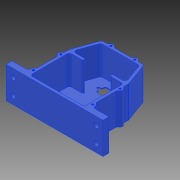
# Autodesk Inventor part: Cam.case.Back
Saved by Autodesk Inventor 2011 (Build 150239000, 239)
## iProperties
Created: 2011-03-29
Part Number: Cam.case.Back
Document SubType Name: Modeling
Designer: Rob
Density: 2.71 g/cm^3
Material: Aluminum-6061
Mass: 146.728 g
Surface Area: 368.166 cm^2
Volume: 54.143 cm^3
Author: Rob
Autodesk Inventor part; units mm, degrees
ref_plane "YZ Plane" through (0, 0, 0) normal (1, 0, 0) x (0, 1, 0)
ref_plane "XZ Plane" through (0, 0, 0) normal (0, 1, 0) x (-1, 0, 0)
ref_plane "XY Plane" through (0, 0, 0) normal (0, 0, 1) x (1, 0, 0)
sketch "Sketch1" plane through (0, 0, 0) normal (0, 0, 1) x (1, 0, 0)
  line L0 (0, 0) -> (0, 80.3)
  line L1 (-56.81, 0) -> (-56.81, 7)
  line L2 (-56.81, 7) -> (-34.81, 7)
  line L3 (0, 0) -> (-56.81, 0)
  line L4 (-34.81, 7) -> (-34.81, 52.2)
  line L5 (0, 80.3) -> (-24.7, 80.3)
  line L6 (-24.7, 80.3) -> (-34.81, 52.2)
  line L7 (0, 77.3) -> (-22.5911, 77.3)
  line L8 (-31.6217, 52.2) -> (-22.5911, 77.3)
  line L9 (-31.6217, 52.2) -> (0, 52.2)
  line L10 (-31.81, 49.2) -> (-31.81, 3)
  line L11 (0, 49.2) -> (-31.81, 49.2)
  line L12 (0, 3) -> (-31.81, 3)
  line L13 (56.81, 0) -> (56.81, 7)
  line L14 (56.81, 7) -> (34.81, 7)
  line L15 (0, 0) -> (56.81, 0)
  line L16 (34.81, 7) -> (34.81, 52.2)
  line L17 (0, 80.3) -> (24.7, 80.3)
  line L18 (24.7, 80.3) -> (34.81, 52.2)
  line L19 (0, 77.3) -> (22.5911, 77.3)
  line L20 (31.6217, 52.2) -> (22.5911, 77.3)
  line L21 (31.6217, 52.2) -> (0, 52.2)
  line L22 (31.81, 49.2) -> (31.81, 3)
  line L23 (0, 49.2) -> (31.81, 49.2)
  line L24 (0, 3) -> (31.81, 3)
  circle A0 centre (-34.81, 10) radius 3
  circle A1 centre (-34.81, 42.2) radius 3
  circle A2 centre (34.81, 42.2) radius 3
  circle A3 centre (34.81, 10) radius 3
  circle A4 centre (-14, 80.3) radius 3
  circle A5 centre (14, 80.3) radius 3
  dimension "d2" = 7
  dimension "d3" = 22
  dimension "d5" = 45.2
  dimension "d6" = 56.81
  dimension "d7" = 24.7
  dimension "d8" = 28.1
  dimension "d10" = 3
  dimension "d12" = 3
  dimension "d13" = 25.1
  dimension "d14" = 3
  dimension "d15" = 3
  dimension "d16" = 3
  dimension "d19" = 6
  dimension "d20" = 6
  dimension "d21" = 6
  dimension "d22" = 6
  dimension "d23" = 10
  dimension "d24" = 10
  dimension "d25" = 10
  dimension "d26" = 10
  dimension "d27" = 6
  dimension "d28" = 6
  dimension "d29" = 14
  dimension "d30" = 14
  constraints: 52 end point, 10 point on line, 9 symmetric about line, 6 centre point, 6 perpendicular, 5 parallel, 1 vertical
  measures "d2" distance of L1.start L1.end
  measures "d3" distance of L1.end L2.end
  measures "d5" distance of L2.end L4.end
  measures "d6" distance of L0.start L1.start
  measures "d7" distance of L0.end L5.end
  measures "d8" vertical distance of L5.end L4.end
  measures "d10" distance between parallel lines of L5 L7
  measures "d12" distance between parallel lines of L6 L8
  measures "d13" distance between parallel lines of L7 L9
  measures "d14" distance between parallel lines of L11 L9
  measures "d15" distance between parallel lines of L4 L10
  measures "d16" distance between parallel lines of L3 L12
  measures "d19" diameter of A0
  measures "d20" diameter of A1
  measures "d21" diameter of A2
  measures "d22" diameter of A3
  measures "d23" distance from line of L3 A0.centre
  measures "d24" distance from line of L9 A1.centre
  measures "d25" distance from line of L21 A2.centre
  measures "d26" distance from line of L15 A3.centre
  measures "d27" diameter of A4
  measures "d28" diameter of A5
  measures "d29" distance from line of L0 A4.centre
  measures "d30" distance from line of L0 A5.centre
extrude "Extrusion1" add sketch "Sketch1" along normal blind 37
sketch "Sketch2" plane through (0, 0, 37) normal (0, 0, 1) x (1, 0, 0)
  line L0 (0, 0) -> (0, 80.3)
  line L1 (-56.81, 0) -> (-56.81, 7)
  line L2 (-56.81, 7) -> (-34.81, 7)
  line L3 (0, 0) -> (-56.81, 0)
  line L4 (-34.81, 7) -> (-34.81, 52.2)
  line L5 (0, 80.3) -> (-24.7, 80.3)
  line L6 (-24.7, 80.3) -> (-34.81, 52.2)
  line L7 (0, 77.3) -> (-22.5911, 77.3)
  line L8 (-31.6217, 52.2) -> (-22.5911, 77.3)
  line L9 (-31.6217, 52.2) -> (0, 52.2)
  line L10 (-31.81, 49.2) -> (-31.81, 3)
  line L11 (0, 49.2) -> (-31.81, 49.2)
  line L12 (0, 3) -> (-31.81, 3)
  line L13 (34.81, 7) -> (34.81, 52.2)
  line L14 (31.81, 49.2) -> (31.81, 3)
  line L15 (56.81, 7) -> (34.81, 7)
  line L16 (56.81, 0) -> (56.81, 7)
  line L17 (31.6217, 52.2) -> (22.5911, 77.3)
  line L18 (24.7, 80.3) -> (34.81, 52.2)
  line L19 (0, 80.3) -> (24.7, 80.3)
  line L20 (0, 77.3) -> (22.5911, 77.3)
  line L21 (31.6217, 52.2) -> (0, 52.2)
  line L22 (0, 49.2) -> (31.81, 49.2)
  line L23 (0, 3) -> (31.81, 3)
  line L24 (0, 0) -> (56.81, 0)
  circle A0 centre (-34.81, 10) radius 3
  circle A1 centre (-34.81, 42.2) radius 3
  circle A2 centre (34.81, 42.2) radius 3
  circle A3 centre (34.81, 10) radius 3
  circle A4 centre (-14, 80.3) radius 3
  circle A5 centre (14, 80.3) radius 3
  dimension "d31" = 7
  dimension "d32" = 22
  dimension "d33" = 45.2
  dimension "d34" = 56.81
  dimension "d35" = 24.7
  dimension "d36" = 28.1
  dimension "d37" = 3
  dimension "d38" = 3
  dimension "d39" = 25.1
  dimension "d40" = 3
  dimension "d41" = 3
  dimension "d42" = 3
  dimension "d43" = 6
  dimension "d44" = 6
  dimension "d45" = 6
  dimension "d46" = 6
  dimension "d47" = 10
  dimension "d48" = 10
  dimension "d49" = 10
  dimension "d50" = 10
  dimension "d51" = 6
  dimension "d52" = 6
  dimension "d53" = 14
  dimension "d54" = 14
  constraints: 52 end point, 10 point on line, 9 symmetric about line, 6 centre point, 6 perpendicular, 5 parallel, 1 vertical
  measures "d31" distance of L1.start L1.end
  measures "d32" distance of L1.end L2.end
  measures "d33" distance of L2.end L4.end
  measures "d34" distance of L0.start L1.start
  measures "d35" distance of L0.end L5.end
  measures "d36" vertical distance of L5.end L4.end
  measures "d37" distance between parallel lines of L5 L7
  measures "d38" distance between parallel lines of L6 L8
  measures "d39" distance between parallel lines of L7 L9
  measures "d40" distance between parallel lines of L11 L9
  measures "d41" distance between parallel lines of L4 L10
  measures "d42" distance between parallel lines of L3 L12
  measures "d43" diameter of A0
  measures "d44" diameter of A1
  measures "d45" diameter of A2
  measures "d46" diameter of A3
  measures "d47" distance from line of L3 A0.centre
  measures "d48" distance from line of L9 A1.centre
  measures "d49" distance from line of L21 A2.centre
  measures "d50" distance from line of L24 A3.centre
  measures "d51" diameter of A4
  measures "d52" diameter of A5
  measures "d53" distance from line of L0 A4.centre
  measures "d54" distance from line of L0 A5.centre
extrude "Extrusion2" cut sketch "Sketch2" against normal blind 34 contours L12 L10 L11 L0 | L0 L22 L14 L23 | L9 L8 L7 L0 | L0 L20 L17 L21
sketch "Sketch3" plane through (0, 0, 0) normal (0, 0, -1) x (-1, 0, 0)
  line L0 (17, 80.3) -> (24.7, 80.3) projected
  line L1 (-11, 80.3) -> (11, 80.3) projected
  line L2 (-34.81, 52.2) -> (-24.7, 80.3) projected
  line L3 (-34.81, 13) -> (-34.81, 39.2) projected
  line L4 (56.81, 0) -> (-56.81, 0) projected
  line L5 (-30.31, 4.5) -> (-1.5, 4.5)
  line L6 (-1.5, 4.5) -> (-1.5, 47.7)
  line L7 (-1.5, 47.7) -> (-30.31, 47.7)
  line L8 (-30.31, 47.7) -> (-30.31, 4.5)
  line L9 (0, 0) -> (0, 103.919)
  line L10 (-30.0276, 52.2) -> (0, 52.2)
  line L11 (-21.5366, 75.8) -> (-30.0276, 52.2)
  line L12 (0, 75.8) -> (-21.5366, 75.8)
  line L13 (30.31, 4.5) -> (1.5, 4.5)
  line L14 (1.5, 4.5) -> (1.5, 47.7)
  line L15 (1.5, 47.7) -> (30.31, 47.7)
  line L16 (30.31, 47.7) -> (30.31, 4.5)
  line L17 (30.0276, 52.2) -> (0, 52.2)
  line L18 (21.5366, 75.8) -> (30.0276, 52.2)
  line L19 (0, 75.8) -> (21.5366, 75.8)
  dimension "d57" = 4.5
  dimension "d59" = 4.5
  dimension "d60" = 1.5
  dimension "d61" = 4.5
  dimension "d62" = 43.2
  dimension "d63" = 4.5
  dimension "d64" = 4.5
  constraints: 32 end point, 6 parallel, 6 symmetric about line, 2 perpendicular, 2 point on line, 1 horizontal
  measures "d57" distance between parallel lines of L4 L5
  measures "d59" distance between parallel lines of L3 L8
  measures "d60" distance between parallel lines of L6 L9
  measures "d61" distance between parallel lines of L7 L10
  measures "d62" distance of L7.end L5.start
  measures "d63" distance between parallel lines of L2 L11
  measures "d64" distance between parallel lines of L12 L1
extrude "Extrusion3" cut sketch "Sketch3" against normal blind 2
sketch "Sketch4" plane through (0, 0, 2) normal (0, 0, -1) x (-1, 0, 0)
  line L0 (21.5366, 75.8) -> (-21.5366, 75.8) projected
  line L1 (-30.0276, 52.2) -> (30.0276, 52.2) projected
  line L2 (-14.1, 64) -> (14.1, 64)
  line L3 (-14.1, 65.5) -> (-10, 65.5)
  line L4 (-10, 65.5) -> (-10, 62.5)
  line L5 (-10, 62.5) -> (-14.1, 62.5)
  line L6 (-14.1, 62.5) -> (-14.1, 65.5)
  line L7 (14.1, 65.5) -> (10, 65.5)
  line L8 (10, 65.5) -> (10, 62.5)
  line L9 (10, 62.5) -> (14.1, 62.5)
  line L10 (14.1, 62.5) -> (14.1, 65.5)
  line L11 (-10, 69.5) -> (10, 69.5)
  line L12 (10, 69.5) -> (10, 58.5)
  line L13 (10, 58.5) -> (-10, 58.5)
  line L14 (-10, 58.5) -> (-10, 69.5)
  line L15 (0, 0) -> (0, 119.5542)
  dimension "d67" = 28.2
  dimension "d68" = 4.1
  dimension "d69" = 3
  dimension "d70" = 4.1
  dimension "d71" = 3
  dimension "d72" = 11
  dimension "d73" = 0
  dimension "d74" = 0
  dimension "d75" = 11.8
  constraints: 28 end point, 8 parallel, 3 horizontal, 3 perpendicular, 2 collinear, 4 other
  measures "d67" distance of L2.start L2.end
  measures "d68" distance of L4.end L5.end
  measures "d69" distance of L3.end L4.end
  measures "d70" distance of L9.end L8.end
  measures "d71" distance of L8.end L7.end
  measures "d72" distance of L11.end L12.end
  measures "d73" distance from line of L10 L2.end
  measures "d74" distance from line of L6 L2.start
  measures "d75" distance between parallel lines of L0 L2
extrude "Extrusion4" cut sketch "Sketch4" against normal blind 2
fillet "Fillet1" radius 1.5 12 edges at (10, 65.5, 2.5) (10, 62.5, 2.5) (14.1, 62.5, 2.5) (10, 58.5, 2.5) (-10, 58.5, 2.5) (-14.1, 62.5, 2.5) (-10, 62.5, 2.5) (-10, 65.5, 2.5) (10, 69.5, 2.5) (-10, 69.5, 2.5) (-14.1, 65.5, 2.5) (14.1, 65.5, 2.5)
fillet "Fillet2" radius 3 16 edges at (34.81, 7, 18.5) (34.81, 13, 18.5) (34.81, 45.2, 18.5) (34.81, 39.2, 18.5) (34.81, 52.2, 18.5) (24.7, 80.3, 18.5) (17, 80.3, 18.5) (11, 80.3, 18.5) (-11, 80.3, 18.5) (-17, 80.3, 18.5) (-24.7, 80.3, 18.5) (-34.81, 52.2, 18.5) (-34.81, 45.2, 18.5) (-34.81, 39.2, 18.5) (-34.81, 7, 18.5) (-34.81, 13, 18.5)
sketch "Sketch5" plane through (0, 0, 37) normal (0, 0, 1) x (1, 0, 0)
  line L0 (-31.81, 49.2) -> (31.81, 49.2) projected
  line L1 (31.6217, 52.2) -> (-31.6217, 52.2) projected
  line L2 (-15.7177, 52.2) -> (15.7177, 52.2)
  line L3 (15.7177, 52.2) -> (15.7177, 49.2)
  line L4 (15.7177, 49.2) -> (-15.7177, 49.2)
  line L5 (-15.7177, 49.2) -> (-15.7177, 52.2)
  line L6 (0, 0) -> (0, 111.6708)
  constraints: 10 end point, 3 parallel, 2 point on line, 1 horizontal, 1 perpendicular, 1 other
extrude "Extrusion5" cut sketch "Sketch5" against normal blind 34
fillet "Fillet3" radius 3 8 edges at (22.5911, 77.3, 20) (31.6217, 52.2, 20) (31.81, 49.2, 20) (31.81, 3, 20) (-31.81, 3, 20) (-31.81, 49.2, 20) (-31.6217, 52.2, 20) (-22.5911, 77.3, 20)
fillet "Fillet4" radius 1.5 4 edges at (-15.7177, 52.2, 20) (-15.7177, 49.2, 20) (15.7177, 49.2, 20) (15.7177, 52.2, 20)
fillet "Fillet5" radius 6 12 edges at (-30.31, 4.5, 1) (-1.5, 4.5, 1) (1.5, 4.5, 1) (30.31, 4.5, 1) (30.0276, 52.2, 1) (21.5366, 75.8, 1) (30.31, 47.7, 1) (1.5, 47.7, 1) (-1.5, 47.7, 1) (-30.31, 47.7, 1) (-21.5366, 75.8, 1) (-30.0276, 52.2, 1)
sketch "Sketch6" plane through (0, 0, 37) normal (0, 0, 1) x (1, 0, 0)
  arc A0 (-36.31, 44.7981) -> (-36.31, 39.6019) centre (-34.81, 42.2) ccw projected
  arc A1 (-36.31, 12.5981) -> (-37.81, 10) centre (-34.81, 10) ccw projected
  arc A2 (37.81, 10) -> (36.31, 12.5981) centre (34.81, 10) ccw projected
  arc A3 (36.31, 39.6019) -> (36.31, 44.7981) centre (34.81, 42.2) ccw projected
  arc A4 (16.5981, 81.8) -> (11.4019, 81.8) centre (14, 80.3) ccw projected
  arc A5 (-11.4019, 81.8) -> (-16.5981, 81.8) centre (-14, 80.3) ccw projected
  point P0 (0, 0)
hole "Hole1" at (-14, 80.3, 37) at (14, 80.3, 37) at (34.81, 42.2, 37) at (34.81, 10, 37) at (-34.81, 42.2, 37) at (-34.81, 10, 37) direction (0, 0, -1) diameter 2.459 depth 8 tip angle 118 thread size "M3x0.5" class "6H" standard "ANSI Metric M Profile"
sketch "Sketch7" plane through (-56.81, 7, 37) normal (0, 1, 0) x (1, 0, 0)
  line L0 (16, 37) -> (0, 37) projected
  line L1 (0, 0) -> (16, 0) projected
  line L2 (56.81, 37) -> (56.81, -24.997)
  circle A0 centre (8, 27.75) radius 4.6705
  circle A1 centre (8, 9.25) radius 2.7794
  circle A2 centre (105.62, 27.75) radius 4.6705
  circle A3 centre (105.62, 9.25) radius 2.7794
  dimension "d92" = 18.5
  dimension "d93" = 37
  dimension "d94" = 9.25
  constraints: 4 centre point, 2 end point, 2 symmetric about line, 1 perpendicular, 2 other
  measures "d92" distance of A1.centre A0.centre
  measures "d93" distance of L0.end L1.start
  measures "d94" distance from line of A0.centre L0
hole "Hole2" at (-48.81, 7, 9.25) at (-48.81, 7, 27.75) at (48.81, 7, 9.25) at (48.81, 7, 27.75) direction (0, -1, 0) diameter 5.5 depth 8 tip angle 118 clearance for "Flat Head Machine Screw" size "M5" standard "Ansi Metric M Profile"
equation "\"d92\" = 2 * d94"
equation "\"d94\" = 0.25 * d93"
body "Solid1"
